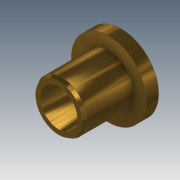
# Autodesk Inventor part: GFM-0608-10_Brass
Saved by Autodesk Inventor 2018 (Build 220112000, 112)
## iProperties
Created: 2017-04-04
Part Number: GFM-0608-10_Brass
Material: Brass
Document SubType Name: Modeling
Designer: NicK Foo
Density: 8.49 g/cm^3
Appearance: Brass - Polished
Author: NicK Foo
Autodesk Inventor part; units mm, degrees
ref_plane "YZ Plane" through (0, 0, 0) normal (1, 0, 0) x (0, 1, 0)
ref_plane "XZ Plane" through (0, 0, 0) normal (0, 1, 0) x (-1, 0, 0)
ref_plane "XY Plane" through (0, 0, 0) normal (0, 0, 1) x (1, 0, 0)
sketch "Sketch1" plane through (0, 0, 0) normal (0, 0, 1) x (1, 0, 0)
  circle A0 centre (0, 0) radius 6
  circle A1 centre (0, 0) radius 3 construction
  circle A2 centre (0, 0) radius 4
  dimension "dia_Flange" = 12
  dimension "dia_Shaft" = 6
  dimension "dia_Outer" = 8
  constraints: 3 centre point, 3 coincident
  measures "dia_Flange" diameter of A0
  measures "dia_Shaft" diameter of A1
  measures "dia_Outer" diameter of A2
extrude "Extrusion1" add sketch "Sketch1" along normal blind 2 contours A0 | A2
extrude "Extrusion2" add sketch "Sketch1" along normal blind 10 contours A2
chamfer "Chamfer1" distance 0.5 angle 30 1 edges at (-4, 0, 10) measured on face at (3.9482, 0.6416, 4.6667)
hole "Hole1" at (0, 0, 0) direction (0, 0, 1) diameter 6 end through all
equation "\"d10\" = dia_Shaft"
body "Solid1"
